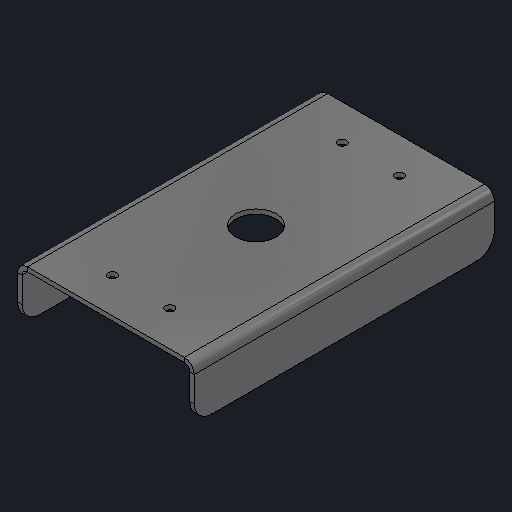
# Autodesk Inventor part: Gooseneck Model-1 Sheet-1
Saved by Autodesk Inventor 2025.1 (Build 291241000, 241)
## iProperties
RuleStatus: InUse
Created: 2026-02-16
Part Number: Gooseneck Model-1 Sheet-1
User Status: Released
Material: SS304
Document SubType Name: Sheet Metal
Designer: Desktop -24
Density: 7.99949 g/cm^3
Sheet Metal Rule: 1/4"
Appearance: Semi-Polished(1)
AfterDocNew0: Mat. Selection
encoded128: ÌStandard Î
encoded39: *STANDARD*
Family: SS304
Author: Desktop -24
Revision Number: 0
Autodesk Inventor part; units mm, degrees
ref_plane "YZ Plane" through (0, 0, 0) normal (1, 0, 0) x (0, 1, 0)
ref_plane "XZ Plane" through (0, 0, 0) normal (0, 1, 0) x (-1, 0, 0)
ref_plane "XY Plane" through (0, 0, 0) normal (0, 0, 1) x (1, 0, 0)
sketch "Sketch4" plane through (0, 0, 0) normal (0, 1, 0) x (-1, 0, 0)
  line L0 (-127, 215.9) -> (127, 215.9)
  line L1 (127, 215.9) -> (127, -215.9)
  line L2 (127, -215.9) -> (-127, -215.9)
  line L3 (-127, -215.9) -> (-127, 215.9)
  line L4 (-127, 215.9) -> (127, -215.9) construction
  line L5 (127, 215.9) -> (-127, -215.9) construction
  point P0 (0, 0)
  dimension "d6" = 431.8
  dimension "d7" = 254
  measures "d6" distance of L0.end L1.end
  measures "d7" distance of L1.end L2.end
extrude "Plate1" add sketch "Sketch4" against normal blind 6.35
sketch "Sketch5" plane through (120.65, 0, -215.9) normal (1, 0, 0) x (0, -1, 0)
  line L0 (0, 431.8) -> (0, 0)
  line L1 (0, 0) -> (76.2, 0)
  line L2 (76.2, 0) -> (76.2, 431.8)
  line L3 (76.2, 431.8) -> (0, 431.8)
  constraints: 6 end point, 1 horizontal, 1 perpendicular, 1 vertical
edge flange "Flange1" height 76.2 angle 90 thickness 6.35 bend radius 7.9502 thickness toward (1, 0, 0) relief tear relief width 6.35 relief depth 3.175 corner gap 6.35 corner form 0 edges at (127, 0, 0) (-127, 0, 0) wall of the first edge with corners at (120.65, 0, 215.9) (120.65, 0, -215.9) (120.65, -76.2, -215.9) (120.65, -76.2, 215.9)
bend "Bend1"
corner "Corner1"
sketch "Sketch6" plane through (0, 0, 0) normal (0, 1, 0) x (1, 0, 0)
  circle A0 centre (0, 0) radius 29.083
  dimension "d19" = 58.166
  constraints: 1 centre point, 1 coincident
  measures "d19" diameter of A0
extrude "Cut1" cut sketch "Sketch6" against normal blind 6.35
sketch "Sketch7" plane through (0, 0, 0) normal (0, 1, 0) x (1, 0, 0)
  line L0 (-41.275, -165.1) -> (41.275, -165.1)
  line L1 (41.275, -165.1) -> (41.275, 165.1)
  line L2 (41.275, 165.1) -> (-41.275, 165.1)
  line L3 (-41.275, 165.1) -> (-41.275, -165.1)
  line L4 (-41.275, -165.1) -> (41.275, 165.1) construction
  line L5 (41.275, -165.1) -> (-41.275, 165.1) construction
  line L6 (112.6998, 215.9) -> (-112.6998, 215.9) projected
  point P0 (0, 0)
  dimension "d22" = 82.55
  dimension "d23" = 50.8
  constraints: 12 end point, 2 midpoint, 2 parallel, 1 horizontal, 1 perpendicular
  measures "d22" distance of L1.end L2.end
  measures "d23" distance between parallel lines of L2 L6
hole "Hole1" at (-41.275, 0, 165.1) at (41.275, 0, 165.1) at (-41.275, 0, -165.1) at (41.275, 0, -165.1) direction (0, -1, 0) diameter 12.7 depth 6.35
fillet "Corner Round1" radius 25.4 4 edges at (-123.825, -76.2, 215.9) (123.825, -76.2, 215.9) (123.825, -76.2, -215.9) (-123.825, -76.2, -215.9)
equation "\"d20\" = Thickness"
equation "\"d29\" = Thickness"
equation "\"d8\" = Thickness"
equation "\"d9\" = BendReliefWidth"
equation "\"d10\" = BendReliefDepth"
equation "\"d11\" = MinimumRemnant"
equation "\"d12\" = TransitionRadius"
equation "\"d15\" = BendRadius"
equation "\"d16\" = CornerReliefSize"
equation "\"d17\" = GapSize"
equation "\"d18\" = JacobiRadiusSize"
equation "\"BendReliefWidth\" = Thickness"
equation "\"BendReliefDepth\" = 0.5 * Thickness"
equation "\"CornerReliefSize\" = 4 * Thickness"
equation "\"MinimumRemnant\" = 2 * Thickness"
equation "\"TransitionRadius\" = BendRadius"
equation "\"JacobiRadiusSize\" = Thickness"
equation "\"GapSize\" = Thickness"
equation "\"Thickness\" = 6.35"
equation "\"BendRadius\" = 7.9502"
body "Solid4"
